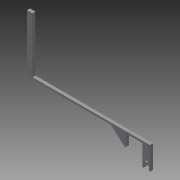
# Autodesk Inventor part: Left Climber Hook
Saved by Autodesk Inventor 2013 (Build 170138000, 138)
## iProperties
Created: 2013-03-16
Part Number: Left Climber Hook
Material: Generic
Document SubType Name: Modeling
Designer: Arpan
Density: 1 g/cm^3
Author: Arpan
Autodesk Inventor part; units mm, degrees
ref_plane "YZ Plane" through (0, 0, 0) normal (1, 0, 0) x (0, 1, 0)
ref_plane "XZ Plane" through (0, 0, 0) normal (0, 1, 0) x (-1, 0, 0)
ref_plane "XY Plane" through (0, 0, 0) normal (0, 0, 1) x (1, 0, 0)
sketch "Sketch1" plane through (0, 0, 0) normal (0, 0, 1) x (1, 0, 0)
  line L0 (0, 0) -> (3.175, 0)
  line L1 (3.175, 0) -> (3.175, 12.7)
  line L2 (3.175, 12.7) -> (22.225, 12.7)
  line L3 (22.225, 12.7) -> (22.225, 0)
  line L4 (22.225, 0) -> (25.4, 0)
  circle A0 centre (12.7, 25.4) radius 4.7815
  line L5 (25.4, 0) -> (25.4, 76.2)
  line L6 (25.4, 76.2) -> (-384.175, 76.2)
  line L7 (0, 69.85) -> (0, 0)
  line L8 (-54.61, 69.85) -> (-54.61, 32.397)
  line L9 (-59.8758, 30.0075) -> (-105.41, 69.85)
  ellipse E0 centre (-26.9408, 50.8) end of major axis (0, 50.8) minor radius 19.05
  arc A1 (-59.8758, 30.0075) -> (-54.61, 32.397) centre (-57.785, 32.397) ccw
  line L10 (-384.175, 69.85) -> (-105.41, 69.85)
  line L11 (-54.61, 69.85) -> (0, 69.85)
  line L12 (-384.175, 69.85) -> (-384.175, 260.35)
  line L13 (-384.175, 260.35) -> (-365.76, 260.35)
  line L14 (-365.76, 260.35) -> (-365.76, 76.2)
  point P0 (-54.61, 25.4)
  dimension "d15" = 26.9408
  dimension "d16" = 19.05
  dimension "d0" = 3.175
  dimension "d1" = 12.7
  dimension "d2" = 19.05
  dimension "d3" = 3.175
  dimension "d4" = 12.7
  dimension "d6" = 9.5631
  dimension "d7" = 12.7
  dimension "d8" = 76.2
  dimension "d9" = 409.575
  dimension "d10" = 6.35
  dimension "d11" = 384.175
  dimension "d13" = 50.8
  dimension "d14" = 54.61
  dimension "d17" = 44.45
  dimension "d18" = 3.175
  dimension "d21" = 190.5
  dimension "d22" = 18.415
  dimension "d24" = 9.525
  dimension "d25" = 184.15
  constraints: 30 end point, 10 perpendicular, 3 horizontal, 3 parallel, 3 point on line, 2 centre point, 2 point on circle, 2 tangent, 2 vertical, 2 other
  measures "d0" distance of L0.start L0.end
  measures "d1" distance of L0.end L1.end
  measures "d2" distance of L1.end L2.end
  measures "d3" distance of L3.end L4.end
  measures "d4" distance of L2.end L3.end
  measures "d6" diameter of A0
  measures "d7" distance from line of L2 A0.centre
  measures "d8" distance of L4.end L5.end
  measures "d9" distance of L5.end L6.end
  measures "d10" distance of L6.end L10.start
  measures "d11" distance of L10.start L7.start
  measures "d13" distance from line of L8 L9.end
  measures "d14" distance between parallel lines of L7 L8
  measures "d17" distance of L8.start point (-54.61, 25.4)
  measures "d18" radius of A1
  measures "d21" distance of L10.start L12.end
  measures "d22" distance of L12.end L13.end
  measures "d24" distance from line of L3 A0.centre
  measures "d25" distance of L13.end L14.end
extrude "Extrusion1" add sketch "Sketch1" along normal blind 9.8425 contours L7 L11 L8 A1 L9 L10 L12 L6 L5 L4 L3 L2 L1 L0 | L6 L12 L13 L14
body "Solid1"
